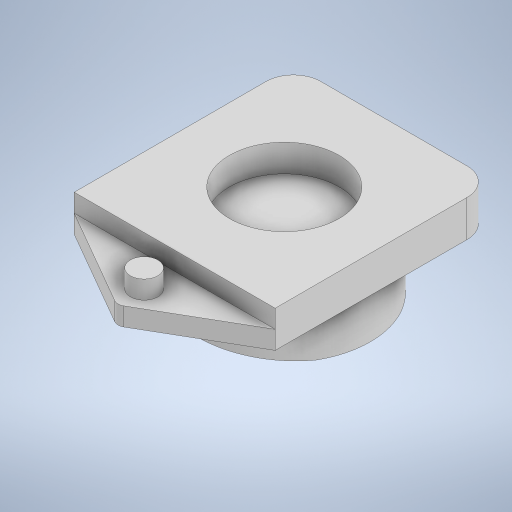
# Autodesk Inventor part: bracket_1
Saved by Autodesk Inventor 2024.3 (Build 283343000, 343)
## iProperties
Created: 2025-10-03
Part Number: bracket_1
Material: 일반
Document SubType Name: Modeling
Designer: joung
Density: 1 g/cm^3
Appearance: 기본값
Author: joung
Autodesk Inventor part; units mm, degrees
ref_plane "YZ Plane" through (0, 0, 0) normal (1, 0, 0) x (0, 1, 0)
ref_plane "XZ Plane" through (0, 0, 0) normal (0, 1, 0) x (-1, 0, 0)
sketch "스케치1" plane through (0, 0, 0) normal (0, 1, 0) x (-1, 0, 0)
  circle A0 centre (0, 0) radius 47
  circle A1 centre (0, 0) radius 35
  line L0 (0, 0) -> (0, 145.5)
  circle A2 centre (0, 145.5) radius 48.5
  circle A3 centre (0, 145.5) radius 36.5
  dimension "d0" = 94
  dimension "d1" = 12
  dimension "d2" = 145.5
  dimension "d3" = 97
  dimension "d4" = 12
  constraints: 4 centre point, 2 coincident, 2 end point, 1 vertical
  measures "d0" diameter of A0
  measures "d1" radial gap between concentric circles of A0 A1
  measures "d2" distance of L0.start L0.end
  measures "d3" diameter of A2
  measures "d4" radial gap between concentric circles of A2 A3
extrude "돌출1" add sketch "스케치1" along normal blind 30 contours A0
sketch "스케치2" plane through (0, 30, 0) normal (0, 1, 0) x (1, 0, 0)
  line L0 (-55, 60) -> (55, 60)
  line L1 (55, 60) -> (55, -60)
  line L2 (55, -60) -> (-55, -60)
  line L3 (-55, -60) -> (-55, 60)
  line L4 (-55, 60) -> (55, -60) construction
  line L5 (55, 60) -> (-55, -60) construction
  point P0 (0, 0)
  dimension "d7" = 110
  dimension "d8" = 120
  constraints: 12 end point, 2 midpoint, 2 parallel, 1 horizontal, 1 perpendicular
  measures "d7" distance of L1.end L2.end
  measures "d8" distance of L0.end L1.end
extrude "돌출2" add sketch "스케치2" along normal blind 20
sketch "스케치3" plane through (0, 30, 0) normal (0, -1, 0) x (1, 0, 0)
  line L0 (-55, 60) -> (55, 60) projected
  line L1 (-55, 60) -> (0, 91.7543)
  line L2 (-55, 60) -> (8.5085, 60) construction
  line L3 (0, 91.7543) -> (55, 60)
  line L4 (55, 60) -> (-55, 60)
  line L5 (0, 91.7543) -> (0, 76.7543)
  circle A0 centre (0, 76.7543) radius 7.5
  point P0 (0, 0)
  dimension "d11" = 30
  dimension "d12" = 15
  dimension "d13" = 15
  dimension "d20" = 30
  constraints: 10 end point, 1 centre point, 1 coincident, 1 collinear, 1 equal length, 1 horizontal, 1 vertical
  measures "d11" angle of L2 L1
  measures "d12" distance of L1.end L5.end
  measures "d13" diameter of A0
  measures "d20" angle of L3 L0
extrude "돌출3" add sketch "스케치3" against normal blind 10 contours L1 L3 L0 | A0
sketch "스케치4" plane through (0, 40, 0) normal (0, 1, 0) x (1, 0, 0)
  line L0 (55, -60) -> (0, -91.7543) projected
  line L1 (0, -91.7543) -> (0, -76.7543)
  circle A0 centre (0, -76.7543) radius 7.5
  point P0 (0, 0)
  dimension "d16" = 15
  dimension "d17" = 15
  constraints: 3 end point, 1 centre point, 1 coincident, 1 vertical
  measures "d16" distance of L0.end L1.end
  measures "d17" diameter of A0
extrude "돌출4" add sketch "스케치4" along normal blind 10
fillet "모깎기1" radius 15 2 edges at (-55, 40, -60) (55, 40, -60)
ref_plane "작업 평면1" through (0, 50, 0) normal (0, 1, 0) x (1, 0, 0)
sketch "스케치6" plane through (0, 50, 0) normal (0, 1, 0) x (1, 0, 0)
  circle A0 centre (0, 0) radius 30
  constraints: 1 centre point, 1 coincident
extrude "돌출6" cut sketch "스케치6" against normal blind 15
fillet "모깎기2" radius 5 1 edges at (0, 35, 91.7543)
sketch "스케치7" plane through (0, 0, 0) normal (0, -1, 0) x (1, 0, 0)
  circle A0 centre (0, 0) radius 35
  constraints: 1 centre point, 1 coincident
extrude "돌출7" add sketch "스케치7" against normal up to surface (30 mm away)
sketch "스케치8" plane through (0, 0, 0) normal (1, 0, 0) x (0, 1, 0)
  line L0 (0, -47) -> (0, 47) projected
  line L1 (0, 0) -> (0, 47)
  line L2 (0, 23.5) -> (2.056, 47)
  line L3 (0, 47) -> (30, 47) projected
  line L4 (0, 23.5) -> (23.5898, 23.5) construction
  line L5 (2.056, 47) -> (0, 47)
  line L6 (0, 0) -> (0, -47)
  line L7 (0, -23.5) -> (0, -47)
  line L8 (0, -47) -> (30, -47) projected
  line L9 (0, -47) -> (0, -47)
  line L10 (0, -23.5) -> (0, -47)
  line L11 (0, -47) -> (0, -47)
  line L12 (0, -23.5) -> (2.056, -47)
  line L13 (0, -23.5) -> (23.5898, -23.5) construction
  line L14 (2.056, -47) -> (0, -47)
  dimension "d31" = 85
  dimension "d32" = 85
  constraints: 24 end point, 4 perpendicular, 4 point on line, 2 equal length, 2 horizontal, 2 midpoint, 1 collinear, 1 vertical
  measures "d31" angle of L4 L2
  measures "d32" angle of L12 L13
extrude "돌출8" cut sketch "스케치8" along normal mid plane 100
